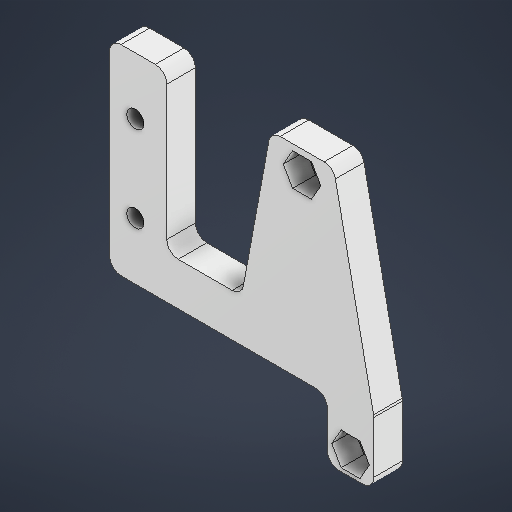
# Autodesk Inventor part: FanMountV2
Saved by Autodesk Inventor 2026.2 (Build 302298000, 298)
## iProperties
Created: 2026-06-02
Part Number: FanMountV2
Material: ABS Plastic
Document SubType Name: Modeling
Designer: gaoet
Density: 1.06 g/cm^3
Appearance: Smooth - White
Author: gaoet
Autodesk Inventor part; units mm, degrees
ref_plane "YZ Plane" through (0, 0, 0) normal (1, 0, 0) x (0, 1, 0)
ref_plane "XZ Plane" through (0, 0, 0) normal (0, 1, 0) x (-1, 0, 0)
ref_plane "XY Plane" through (0, 0, 0) normal (0, 0, 1) x (1, 0, 0)
sketch "Sketch1" plane through (0, 0, 0) normal (0, 0, 1) x (1, 0, 0)
  line L0 (0, 0) -> (10, 0)
  line L1 (10, 0) -> (10, -27.5)
  line L2 (10, -27.5) -> (23.0834, -27.5)
  line L3 (23.0834, -27.5) -> (28.1466, 0)
  line L4 (28.1466, 0) -> (39.1466, 0)
  line L5 (39.1466, 0) -> (46.1888, -34.158)
  line L6 (38.0632, -45.4132) -> (38.0632, -35)
  line L7 (38.0632, -35) -> (0, -35)
  line L8 (0, -35) -> (0, 0)
  line L9 (46.1888, -34.158) -> (46.1888, -45.4132)
  line L10 (46.1888, -45.4132) -> (38.0632, -45.4132)
  line L11 (28.1466, 0) -> (33.3359, 28.1848) construction
  line L12 (33.3359, 28.1848) -> (39.1466, 0) construction
  point P0 (4.5, -10)
  point P1 (4.5, -25)
  point P2 (42.126, -41.9632)
  point P3 (33.6466, -3.9132)
  point P4 (38.0632, -40.2066)
  point P5 (42.126, -45.4132)
  point P6 (33.6466, 0)
  dimension "d0" = 35
  dimension "d1" = 10
  dimension "d2" = 10
  dimension "d3" = 4.5
  dimension "d4" = 100.432
  dimension "d6" = 101.649
  dimension "d7" = 7.5
  dimension "d8" = 15
  dimension "d9" = 8.1256
  dimension "d10" = 38.0632
  dimension "d11" = 10.4132
  dimension "d12" = 3.45
  dimension "d13" = 3.9132
  dimension "d14" = 29.1466
  dimension "d15" = 28.1848
  constraints: 26 end point, 4 perpendicular, 3 midpoint, 3 vertical alignment, 2 collinear, 2 horizontal, 2 vertical, 1 coincident, 1 point on line
  measures "d0" distance between parallel lines of L0 L7
  measures "d1" distance of L0.start L0.end
  measures "d2" distance from line of L0 point (4.5, -10)
  measures "d3" distance from line of L8 point (4.5, -10)
  measures "d4" angle of L2 L3
  measures "d6" angle of L4 L5
  measures "d7" distance between parallel lines of L7 L2
  measures "d8" distance of point (4.5, -25) point (4.5, -10)
  measures "d9" distance from line of L9 point (38.063, -40.207)
  measures "d10" distance between parallel lines of L8 L6
  measures "d11" distance from line of point (42.126, -45.413) L7
  measures "d12" distance from line of L10 point (42.126, -41.963)
  measures "d13" distance of point (33.647, 0) point (33.647, -3.913)
  measures "d14" horizontal distance of point (4.5, -10) point (33.647, -3.913)
  measures "d15" vertical distance of point (33.647, 0) L11.end
extrude "Extrusion1" add sketch "Sketch1" along normal blind 5
hole "Hole1" at (4.5, -10, 0) at (4.5, -25, 0) at (42.126, -41.9632, 0) at (33.6466, -3.9132, 0) direction (0, 0, 1) diameter 3 depth 20
sketch "Sketch2" plane through (0, 0, 5) normal (0, 0, 1) x (1, 0, 0)
  circle A0 centre (33.6466, -3.9132) radius 1.5 projected
  circle A1 centre (42.126, -41.9632) radius 1.5 projected
  circle A2 centre (4.5, -25) radius 1.5 projected
  circle A3 centre (4.5, -10) radius 1.5 projected
  line L0 (0, -35) -> (38.0632, -35) projected
  line L1 (38.0632, -35) -> (38.0632, -45.4132) projected
  line L2 (38.0632, -45.4132) -> (46.1888, -45.4132) projected
  line L3 (46.1888, -45.4132) -> (46.1888, -34.158) projected
  line L4 (46.1888, -34.158) -> (39.1466, 0) projected
  line L5 (39.1466, 0) -> (28.1466, 0) projected
  line L6 (28.1466, 0) -> (23.0834, -27.5) projected
  line L7 (23.0834, -27.5) -> (10, -27.5) projected
  line L8 (10, -27.5) -> (10, 0) projected
  line L9 (10, 0) -> (0, 0) projected
  line L10 (0, 0) -> (0, -35) projected
  line L11 (35.2921, -1.0632) -> (36.9375, -3.9132)
  line L12 (36.9375, -3.9132) -> (35.2921, -6.7632)
  line L13 (35.2921, -6.7632) -> (32.0012, -6.7632)
  line L14 (32.0012, -6.7632) -> (30.3557, -3.9132)
  line L15 (30.3557, -3.9132) -> (32.0012, -1.0632)
  line L16 (32.0012, -1.0632) -> (35.2921, -1.0632)
  line L17 (43.7715, -39.1132) -> (45.4169, -41.9632)
  line L18 (45.4169, -41.9632) -> (43.7715, -44.8132)
  line L19 (43.7715, -44.8132) -> (40.4806, -44.8132)
  line L20 (40.4806, -44.8132) -> (38.8351, -41.9632)
  line L21 (38.8351, -41.9632) -> (40.4806, -39.1132)
  line L22 (40.4806, -39.1132) -> (43.7715, -39.1132)
  dimension "d25" = 6.5818
  dimension "d26" = 6.5818
  constraints: 24 end point, 2 coincident, 2 horizontal, 26 other
  measures "d25" distance of L11.end L14.end
  measures "d26" distance of L17.end L20.end
extrude "Extrusion2" cut sketch "Sketch2" against normal blind 4 contours L11 L12 L13 L14 L15 L16 | L17 L18 L19 L20 L21 L22
fillet "Fillet1" radius 2 11 edges at (0, 0, 2.5) (10, 0, 2.5) (10, -27.5, 2.5) (23.0834, -27.5, 2.5) (28.1466, 0, 2.5) (39.1466, 0, 2.5) (0, -35, 2.5) (38.0632, -35, 2.5) (38.0632, -45.4132, 2.5) (46.1888, -45.4132, 2.5) (46.1888, -34.158, 2.5)
body "Solid1"
